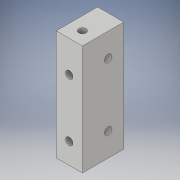
# Autodesk Inventor part: CupHolderBack
Saved by Autodesk Inventor 2019 (Build 230136000, 136)
## iProperties
Created: 2020-12-31
Part Number: CupHolderBack
Material: Типовые
Document SubType Name: Modeling
Designer: Professional
Density: 1 g/cm^3
Appearance: По умолчанию
Author: Professional
Autodesk Inventor part; units mm, degrees
ref_plane "YZ Plane" through (0, 0, 0) normal (1, 0, 0) x (0, 1, 0)
ref_plane "XZ Plane" through (0, 0, 0) normal (0, 1, 0) x (-1, 0, 0)
ref_plane "XY Plane" through (0, 0, 0) normal (0, 0, 1) x (1, 0, 0)
sketch "Эскиз1" plane through (0, 0, 0) normal (0, 1, 0) x (-1, 0, 0)
  line L0 (0, 0) -> (-10, 0)
  line L1 (-10, 0) -> (-10, -15.8)
  line L2 (-10, -15.8) -> (0, -15.8)
  line L3 (0, -15.8) -> (0, 0)
  dimension "d0" = 10
  dimension "d1" = 15.8
  constraints: 8 end point, 2 parallel, 1 horizontal, 1 perpendicular
  measures "d0" distance between parallel lines of L3 L1
  measures "d1" distance between parallel lines of L2 L0
extrude "Выдавливание1" add sketch "Эскиз1" along normal blind 42
sketch "Эскиз2" plane through (10, 0, -15.8) normal (0, 0, -1) x (-1, 0, 0)
  line L0 (0, 0) -> (10, 0) projected
  line L1 (0, 42) -> (10, 42) projected
  point P0 (5, 5)
  point P1 (5, 37)
  point P2 (5, 0)
  dimension "d32" = 5
  dimension "d33" = 5
  constraints: 2 vertical alignment, 1 midpoint
  measures "d32" distance from line of L1 point (5, 37)
  measures "d33" distance from line of L0 point (5, 5)
hole "Отверстие1" at (5, 5, -15.8) at (5, 37, -15.8) direction (0, 0, 1) diameter 2.8 depth 8
sketch "Эскиз3" plane through (10, 0, 0) normal (1, 0, 0) x (0, 0, -1)
  line L0 (0, 42) -> (15.8, 42) projected
  line L1 (0, 0) -> (15.8, 0) projected
  line L2 (15.8, 0) -> (15.8, 42) projected
  point P0 (9.8, 33)
  point P1 (9.8, 9)
  point P2 (7.9, 42)
  dimension "d34" = 9
  dimension "d35" = 9
  dimension "d37" = 6
  constraints: 1 vertical alignment
  measures "d34" distance from line of L0 point (9.8, 33)
  measures "d35" distance from line of L1 point (9.8, 9)
  measures "d37" distance from line of L2 point (9.8, 33)
hole "Отверстие2" at (10, 33, -9.8) at (10, 9, -9.8) direction (-1, 0, 0) diameter 2.8 end through all
sketch "Эскиз7" plane through (0, 42, 0) normal (0, 1, 0) x (1, 0, 0)
  line L0 (0, 0) -> (10, 0) projected
  point P0 (5, 5)
  point P1 (5, 0)
  dimension "d45" = 5
  constraints: 1 midpoint, 1 vertical alignment
  measures "d45" distance from line of L0 point (5, 5)
hole "Отверстие5" at (5, 42, -5) direction (0, -1, 0) diameter 2.8 depth 8
sketch "Эскиз9" plane through (0, 0, 0) normal (0, 0, 1) x (1, 0, 0)
  line L0 (0, 42) -> (10, 42) projected
  line L1 (0, 0) -> (10, 0) projected
  point P0 (5, 30)
  point P1 (5, 8)
  point P2 (5, 42)
  dimension "d53" = 12
  dimension "d54" = 8
  constraints: 2 vertical alignment, 1 midpoint
  measures "d53" distance from line of L0 point (5, 30)
  measures "d54" distance from line of L1 point (5, 8)
hole "Отверстие6" at (5, 30, 0) at (5, 8, 0) direction (0, 0, -1) diameter 2.8 depth 8
